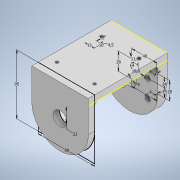
# Autodesk Inventor part: Holder2
Saved by Autodesk Inventor 2020 (Build 240168000, 168)
## iProperties
Created: 2020-06-15
Part Number: Holder2
Material: Generic
Document SubType Name: Modeling
Designer: jurre
Density: 1 g/cm^3
Appearance: Default
Author: jurre
Autodesk Inventor part; units mm, degrees
ref_plane "YZ Plane" through (0, 0, 0) normal (1, 0, 0) x (0, 1, 0)
ref_plane "XZ Plane" through (0, 0, 0) normal (0, 1, 0) x (-1, 0, 0)
ref_plane "XY Plane" through (0, 0, 0) normal (0, 0, 1) x (1, 0, 0)
sketch "Sketch1" plane through (0, 0, 0) normal (0, 1, 0) x (-1, 0, 0)
  line L0 (45, 50.5) -> (-45, 50.5)
  line L1 (-45, 50.5) -> (-45, -50.5)
  line L2 (-45, -50.5) -> (45, -50.5)
  line L3 (45, -50.5) -> (45, 50.5)
  line L4 (45, 50.5) -> (-45, -50.5) construction
  line L5 (-45, 50.5) -> (45, -50.5) construction
  point P0 (0, 0)
  dimension "d0" = 90
  dimension "d1" = 101
  constraints: 12 end point, 2 midpoint, 2 parallel, 1 horizontal, 1 perpendicular
  measures "d0" distance of L0.start L0.end
  measures "d1" distance of L2.end L0.start
extrude "Extrusion1" add sketch "Sketch1" along normal blind 10
sketch "Sketch2" plane through (-45, 0, 50.5) normal (0, 0, 1) x (1, 0, 0)
  line L0 (90, 10) -> (0, 10) projected
  line L1 (0, 10) -> (90, 10)
  line L2 (90, 10) -> (90, -85)
  line L3 (90, -85) -> (0, -85)
  line L4 (0, -85) -> (0, 10)
  circle A0 centre (45, -40) radius 45
  circle A1 centre (45, -40) radius 11
  point P0 (45, 0)
  point P1 (0, -40)
  point P2 (90, -40)
  dimension "d4" = 90
  dimension "d5" = 95
  dimension "d10" = 22
  constraints: 8 end point, 3 tangent, 2 centre point, 2 parallel, 1 coincident, 1 horizontal, 1 perpendicular
  measures "d4" distance of L2.end L3.end
  measures "d5" distance of L3.end L0.end
  measures "d10" diameter of A1
extrude "Extrusion2" add sketch "Sketch2" along normal blind 10 contours L2 A0 L4 L0 | A0
extrude "Extrusion4" add sketch "Sketch2" against normal blind 14.5 from surface at -101 contours L2 A0 L4 L0 | A0
sketch "Sketch3" plane through (0, -40, -65) normal (0, 0, -1) x (-1, 0, 0)
  circle A0 centre (0, 0) radius 9.4
  circle A1 centre (11.05, 14) radius 2
  circle A2 centre (11.05, -14) radius 2
  circle A3 centre (-28.95, 14) radius 2
  circle A4 centre (-28.95, -14) radius 2
  circle A5 centre (0, 0) radius 8.9
  line L0 (-45, 50) -> (45, 50) projected
  point P0 (0, 40)
  dimension "d13" = 18.8
  dimension "d14" = 4
  dimension "d15" = 4
  dimension "d16" = 28
  dimension "d17" = 11.05
  dimension "d18" = 14
  dimension "d19" = 4
  dimension "d20" = 4
  dimension "d21" = 40
  dimension "d22" = 40
  dimension "d23" = 14
  dimension "d24" = 28
  dimension "d25" = 14
  dimension "d30" = 0.5
  constraints: 6 centre point
  measures "d13" diameter of A0
  measures "d14" diameter of A1
  measures "d15" diameter of A2
  measures "d16" distance of A1.centre A2.centre
  measures "d17" horizontal distance of A1.centre A0.centre
  measures "d18" vertical distance of A1.centre A0.centre
  measures "d19" diameter of A3
  measures "d20" diameter of A4
  measures "d21" distance of A3.centre A1.centre
  measures "d22" distance of A4.centre A2.centre
  measures "d23" vertical distance of A4.centre A0.centre
  measures "d24" distance of A3.centre A4.centre
  measures "d25" vertical distance of A0.centre A3.centre
  measures "d30" radial gap between concentric circles of A0 A5
sketch "Sketch4" plane through (0, -40, -50.5) normal (0, 0, 1) x (1, 0, 0)
  circle A0 centre (28.95, 14) radius 2 projected
  circle A1 centre (28.95, -14) radius 2 projected
  circle A2 centre (-11.05, -14) radius 2 projected
  circle A3 centre (-11.05, 14) radius 2 projected
  point P0 (0, 40)
hole "Hole2" at (-11.05, -54, -50.5) at (-11.05, -26, -50.5) at (28.95, -54, -50.5) at (28.95, -26, -50.5) direction (0, 0, -1) diameter 3.242 depth 14.5 tip angle 118 counterbore diameter 8 counterbore depth 4 thread size "M4x0.7" class "6H" standard "ISO Metric profile"
thread "Thread2" size "M4x0.7" class "6H" standard "ANSI Metric M Profile" full length
thread "Thread3" size "M4x0.7" class "6H" standard "ANSI Metric M Profile" full length
thread "Thread4" size "M4x0.7" class "6H" standard "ANSI Metric M Profile" full length
thread "Thread5" size "M4x0.7" class "6H" standard "ANSI Metric M Profile" full length
sketch "Sketch5" plane through (0, 0, 0) normal (0, -1, 0) x (1, 0, 0)
  circle A0 centre (-30, -35.5) radius 5
  line L0 (-45, -50.5) -> (-45, 50.5) projected
  line L1 (-45, 0) -> (45, 0)
  line L2 (45, -65) -> (45, 60.5) projected
  line L3 (-45, 50.5) -> (45, 50.5) projected
  line L4 (0, 50.5) -> (0, -50.5)
  line L5 (45, -50.5) -> (-45, -50.5) projected
  circle A1 centre (-30, -35.5) radius 2.25
  circle A2 centre (-30, 35.5) radius 5
  circle A3 centre (-30, 35.5) radius 2.25
  circle A4 centre (30, -35.5) radius 5
  circle A5 centre (30, -35.5) radius 2.25
  circle A6 centre (30, 35.5) radius 2.25
  circle A7 centre (30, 35.5) radius 5
  point P0 (0, 0)
  dimension "d59" = 10
  dimension "d60" = 15
  dimension "d61" = 15
  dimension "d62" = 4.5
  constraints: 8 centre point, 6 symmetric about line, 4 coincident, 4 end point, 3 midpoint, 1 horizontal, 1 point on line, 6 other
  measures "d59" diameter of A0
  measures "d60" distance from line of L0 A0.centre
  measures "d61" distance from line of L5 A0.centre
  measures "d62" diameter of A1
extrude "Extrusion6" cut sketch "Sketch5" against normal blind 2 contours A0 | A2 | A4 | A7
extrude "Extrusion7" cut sketch "Sketch5" against normal through all contours A1 | A3 | A5 | A6
sketch "Sketch6" plane through (45, -40, 60.5) normal (1, 0, 0) x (0, 0, -1)
  line L0 (7.6158, 13.5) -> (-7.6158, 13.5)
  line L1 (125.5, 0) -> (139, 0)
  line L2 (125.5, 0) -> (111, 0) projected
  line L3 (125.5, -11) -> (125.5, 11) projected
  circle A0 centre (139, 0) radius 15.5
  line L4 (125.5, 50) -> (125.5, 0) projected
  line L5 (125.5, 7.6158) -> (125.5, -7.6158)
  point P0 (60.5, 40)
  constraints: 6 end point, 2 point on circle, 2 point on line, 1 centre point, 1 coincident, 1 horizontal
extrude "Extrusion8" cut sketch "Sketch6" against normal blind 20
chamfer "Chamfer1" distance 4 angle 45 2 edges at (0, 0, -50.5) (0, 0, 50.5)
body "Solid1"
